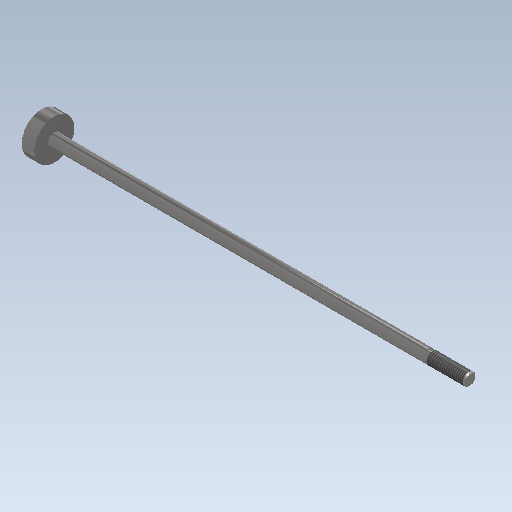
# Autodesk Inventor part: CJ2B16-125Z_ROD
Saved by Autodesk Inventor 2021.2 (Build 252289000, 289)
## iProperties
Part Number: CJ2B16-125Z_ROD
Material: ステンレス鋼
Catalog Web Link: www.cadenas.de
Description: CJ2-Z ROD-Air Cylinder/Standard: Double Acting Single Rod
Vendor: SMC
Document SubType Name: Modeling
Designer: partserver
Manufacturer: SMC
Mass: 33.9505 g
Surface Area: 32.5664 cm^2
Volume: 4.24381 cm^3
Density: 8 g/cm^3
Appearance: 半つや出し
Category: PARTsolutions
Company: SMC
PSOL_IDENT_0: {$CADENAS_DATA\23d-libs\smc_jp\actuator\standard_air_cylinder\cj2\cj2_z\parts\cj2_z_rod.prj},199 {VT
PSOL_IDENT_1: YP=3D},{NB=CJ2B16-125Z_ROD},{LINA=CJ2B16-125Z_ROD},{NN=CJ2-Z ROD},{DATE=09.12.2020 03:32:51},{GEOMDA
PSOL_IDENT_2: TE=10.07.2020 06:48:21},{VERSION=},{LINEID=410},{WBVAR=STROKE,CUSHION,RODB},{WBNUMERIC=STROKE}  {NB=
PSOL_IDENT_3: CJ2B16-125Z_ROD},{LINA=CJ2B16-125Z_ROD},{KT=DUMMY},{ORDER=CJ2B16-125Z},{BORE=16},{MOUNT=(B) Basic},{
PSOL_IDENT_4: MOUNTX=B},{STROKE=125},{CUSHION=},{RODB=},{A=15},{D=5},{H=28},{MM=M5x0.8},{MM1=5},{MM2=0.8},{NA=12.5
PSOL_IDENT_5: },{NA1=12.5},{NA2=21.000},{S=47},{S1=47.000},{S2=66.000},{NB1=9.500},{SMAX=400.000},{P=10},{P1=8.000
PSOL_IDENT_6: },{P2=11.000},{P3=10.000}
NB: CJ2B16-125Z_ROD
NN: CJ2-Z ROD
NT: Air Cylinder/Standard: Double Acting Single Rod
NBSYN: $ORDER._ROD
LINA: CJ2B16-125Z_ROD
CATALOG: SMC (JP
BORE: 16
MOUNT: (B) Basic
STROKE: 125
CUSHION: (-) Rubber cushion
RODB: (-) None
A: 15
D: 5
H: 28
MM: M5x0.8
MM1: 5
MM2: 0.8
NA1: 12.5
NA2: 21
S1: 47
S2: 66
NB1: 9.5
SMAX: 400
P1: 8
P2: 11
P3: 10
SUPPLIER: SMC
ARTICLENO: CJ2B16-125Z_ROD
BOMINFO: CJ2B16-125Z_ROD
CREATOR: CADENAS GmbH
Title: CJ2B16-125Z_ROD
Author: Cadenas PARTsolutions
Comments: Air Cylinder/Standard: Double Acting Single Rod
Autodesk Inventor part; units mm, degrees
sketch "Sketch_5" plane through (0, 0, 0) normal (0, 0, 1) x (1, 0, 0)
  line L0 (170.5, 0) -> (0, 0)
  line L1 (0, 0) -> (0, 2.0095)
  line L2 (0, 2.0095) -> (0.4905, 2.5)
  line L3 (0.4905, 2.5) -> (15, 2.5)
  line L4 (15, 2.5) -> (15, 2.067)
  line L5 (15, 2.067) -> (16.5, 2.067)
  line L6 (16.5, 2.067) -> (16.5, 2.5)
  line L7 (16.5, 2.5) -> (165.5, 2.5)
  line L8 (165.5, 2.5) -> (165.5, 8)
  line L9 (165.5, 8) -> (170.5, 8)
  line L10 (170.5, 8) -> (170.5, 0)
  line L11 (170.5, 0) -> (0, 0)
  constraints: 24 end point
revolve "Revolution1" add sketch "Sketch_5" angle 360 about axis through (170.5, 0, 0) along (1, 0, 0)
thread "Thread1" size "M5x0.8" class "6g" standard "ISO Metric profile" full length
ref_plane "ROD_BA_XY" through (10, 0, 0) normal (-1, 0, 0) x (0, 0, -1)
ref_plane "ROD_BA_YZ" through (10, 0, 0) normal (0, 0, -1) x (0, -1, 0)
ref_plane "ROD_BA_ZX" through (10, 0, 0) normal (0, -1, 0) x (-1, 0, 0)
ref_plane "ROD_BODY_XY" through (28, 0, 0) normal (-1, 0, 0) x (0, 0, -1)
ref_plane "ROD_BODY_YZ" through (28, 0, 0) normal (0, 0, -1) x (0, -1, 0)
ref_plane "ROD_BODY_ZX" through (28, 0, 0) normal (0, -1, 0) x (-1, 0, 0)
ref_plane "rodnt1_XY" through (7.5, 0, 0) normal (1, 0, 0) x (0, 0, -1)
ref_plane "rodnt1_YZ" through (7.5, 0, 0) normal (0, 0, -1) x (0, 1, 0)
ref_plane "rodnt1_ZX" through (7.5, 0, 0) normal (0, 1, 0) x (1, 0, 0)
body "Solid1"
